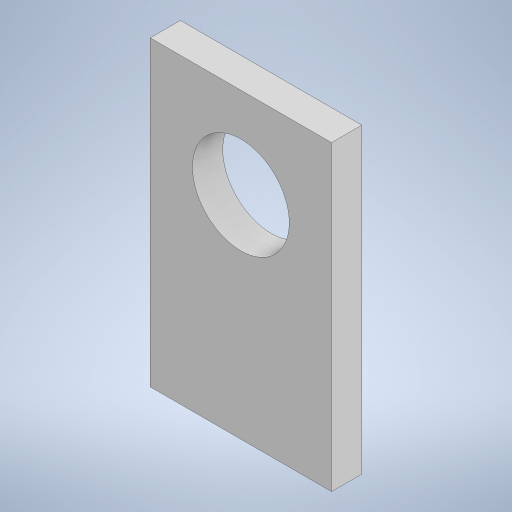
# Autodesk Inventor part: connector2_cooler
Saved by Autodesk Inventor 2023 (Build 270158000, 158)
## iProperties
Created: 2023-06-13
Part Number: connector2_cooler
Material: 一般
Document SubType Name: Sheet Metal
Designer: 310611102
Density: 1 g/cm^3
Sheet Metal Rule: Default_mm
Appearance: 預設
Author: 310611102
Autodesk Inventor part; units mm, degrees
ref_plane "YZ Plane" through (0, 0, 0) normal (1, 0, 0) x (0, 1, 0)
ref_plane "XZ Plane" through (0, 0, 0) normal (0, 1, 0) x (-1, 0, 0)
ref_plane "XY Plane" through (0, 0, 0) normal (0, 0, 1) x (1, 0, 0)
sketch "Sketch1" plane through (0, 0, 0) normal (0, 0, 1) x (1, 0, 0)
  line L0 (-3, 5) -> (3, 5)
  line L1 (3, 5) -> (3, -5)
  line L2 (3, -5) -> (-3, -5)
  line L3 (-3, -5) -> (-3, 5)
  line L4 (-3, 5) -> (3, -5) construction
  line L5 (3, 5) -> (-3, -5) construction
  circle A0 centre (0, 2) radius 1.6
  point P0 (0, 0)
  dimension "d0" = 10
  dimension "d1" = 6
  dimension "d3" = 3.2
  dimension "d4" = 3
  measures "d0" distance of L0.end L1.end
  measures "d1" distance of L0.start L0.end
  measures "d3" diameter of A0
  measures "d4" distance from line of L0 A0.centre
extrude "Plate1" add sketch "Sketch1" along normal blind 1
equation "\"d2\" = 厚度"
equation "\"折彎半徑\" = 厚度"
equation "\"折彎離隙寬度\" = 厚度"
equation "\"折彎離隙深度\" = 0.5 * 厚度"
equation "\"轉角離隙大小\" = 4 * 厚度"
equation "\"最小剩餘\" = 2 * 厚度"
equation "\"轉移半徑\" = 折彎半徑"
equation "\"Jacobi半徑大小\" = 折彎半徑"
equation "\"間隙大小\" = 厚度"
equation "\"厚度\" = 1"
body "Solid1"
